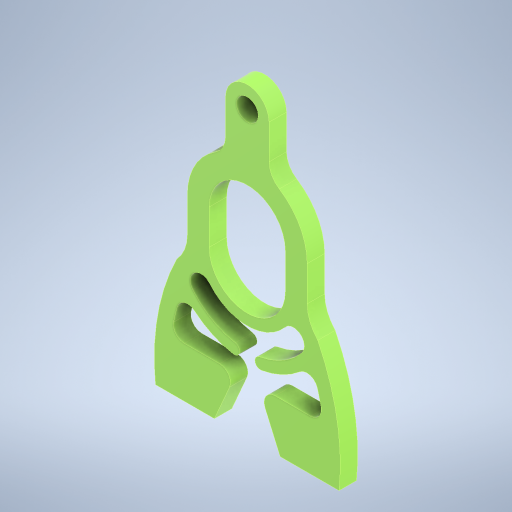
# Autodesk Inventor part: Back distributor
Saved by Autodesk Inventor 2023 (Build 270158000, 158)
## iProperties
Created: 2022-05-02
Part Number: Back distributor
Material: Phenolic Resin
Document SubType Name: Modeling
Designer: Devin
Density: 1.38 g/cm^3
Appearance: Light Green
Author: Devin
Autodesk Inventor part; units mm, degrees
ref_plane "YZ Plane" through (0, 0, 0) normal (1, 0, 0) x (0, 1, 0)
ref_plane "XZ Plane" through (0, 0, 0) normal (0, 1, 0) x (-1, 0, 0)
ref_plane "XY Plane" through (0, 0, 0) normal (0, 0, 1) x (1, 0, 0)
sketch "Sketch1" plane through (0, 0, 0) normal (0, 0, 1) x (1, 0, 0)
  circle A0 centre (0, 0) radius 1.27
  arc A1 (2.54, 0) -> (-2.54, 0) centre (0, 0) ccw
  line L0 (4.445, -12.065) -> (4.445, -16.129)
  line L1 (-4.445, -16.129) -> (-4.445, -12.065)
  arc A2 (-4.445, -16.129) -> (0, -20.574) centre (0, -16.129) ccw
  arc A3 (0, -20.574) -> (4.445, -16.129) centre (0, -16.129) ccw
  arc A4 (4.445, -12.065) -> (0, -7.62) centre (0, -12.065) ccw
  arc A5 (0, -7.62) -> (-4.445, -12.065) centre (0, -12.065) ccw
  arc A6 (-3.7253, -6.1564) -> (-6.985, -12.065) centre (0, -12.065) ccw
  line L2 (-6.985, -12.065) -> (-6.985, -16.129)
  line L3 (6.985, -16.129) -> (6.985, -12.065)
  arc A7 (6.985, -12.065) -> (3.7253, -6.1564) centre (0, -12.065) ccw
  line L4 (2.54, 0) -> (2.54, -4.0078)
  line L5 (-2.54, -4.0078) -> (-2.54, 0)
  arc A8 (-3.7253, -6.1564) -> (-2.54, -4.0078) centre (-5.08, -4.0078) ccw
  arc A9 (2.54, -4.0078) -> (3.7253, -6.1564) centre (5.08, -4.0078) ccw
  line L6 (0, 10.6389) -> (0, -34.9182) construction
  arc A10 (0, -21.844) -> (4.4127, -19.7607) centre (0, -16.129) ccw
  line L7 (5.715, -16.129) -> (5.715, -16.0811)
  arc A11 (-4.4127, -19.7607) -> (0, -21.844) centre (0, -16.129) ccw
  arc A12 (1.4151, -24.2618) -> (6.3739, -21.3748) centre (0, -16.129) ccw
  arc A13 (-6.3739, -21.3748) -> (-1.4151, -24.2618) centre (0, -16.129) ccw
  arc A14 (6.3739, -21.3748) -> (4.4127, -19.7607) centre (5.3933, -20.5678) ccw
  arc A15 (-4.4127, -19.7607) -> (-6.3739, -21.3748) centre (-5.3933, -20.5678) ccw
  arc A16 (-6.1402, -23.4108) -> (-1.6329, -25.513) centre (0, -16.129) ccw
  arc A17 (-1.6329, -25.513) -> (-1.4151, -24.2618) centre (-1.524, -24.8874) ccw
  arc A18 (1.4151, -24.2618) -> (1.6329, -25.513) centre (1.524, -24.8874) ccw
  arc A19 (-8.2215, -19.2053) -> (-6.985, -16.129) centre (-11.43, -16.129) ccw
  arc A20 (-8.2215, -19.2053) -> (-10.7047, -33.133) centre (14.5533, -30.451) ccw
  arc A21 (-8.1811, -24.0368) -> (-8.6001, -25.7693) centre (14.5533, -30.451) ccw
  arc A22 (6.985, -16.129) -> (8.2215, -19.2053) centre (11.43, -16.129) ccw
  arc A23 (10.7047, -33.133) -> (8.2215, -19.2053) centre (-14.5533, -30.451) ccw
  arc A24 (8.6001, -25.7693) -> (8.1811, -24.0368) centre (-14.5533, -30.451) ccw
  arc A25 (1.6329, -25.513) -> (6.1402, -23.4108) centre (0, -16.129) ccw
  line L8 (-3.8359, -33.133) -> (-2.0683, -29.0674)
  line L9 (3.8359, -33.133) -> (2.0683, -29.0674)
  line L10 (-7.3553, -27.291) -> (-3.2329, -27.291)
  line L11 (3.2329, -27.291) -> (7.3553, -27.291)
  line L12 (-10.7047, -33.133) -> (-3.8359, -33.133)
  line L13 (3.8359, -33.133) -> (10.7047, -33.133)
  arc A26 (-6.1402, -23.4108) -> (-8.1811, -24.0368) centre (-6.9589, -24.3817) ccw
  arc A27 (8.1811, -24.0368) -> (6.1402, -23.4108) centre (6.9589, -24.3817) ccw
  arc A28 (7.3553, -27.291) -> (8.6001, -25.7693) centre (7.3553, -26.021) ccw
  arc A29 (-8.6001, -25.7693) -> (-7.3553, -27.291) centre (-7.3553, -26.021) ccw
  arc A30 (-2.0683, -29.0674) -> (-3.2329, -27.291) centre (-3.2329, -28.561) ccw
  arc A31 (3.2329, -27.291) -> (2.0683, -29.0674) centre (3.2329, -28.561) ccw
  point P0 (4.445, -20.574)
  point P1 (4.445, -7.62)
  point P2 (-4.445, -20.574)
  point P3 (-2.54, -2.0039)
  point P4 (5.7149, -19.3392)
  point P5 (-5.7151, -19.3392)
  point P6 (-0.889, -24.8874)
  point P7 (0.889, -24.8874)
  point P8 (-10.7948, -28.8286)
  point P9 (10.7948, -28.8286)
  point P10 (-8.8563, -27.291)
  point P11 (8.8563, -27.291)
  point P12 (1.524, -25.5224)
  point P13 (-1.2959, -27.291)
  point P14 (1.2959, -27.291)
  point P15 (-4.4127, -19.7607)
  point P16 (0, -7.62)
  point P17 (0, -20.574)
  dimension "d0" = 2.54
  dimension "d1" = 1.27
  dimension "d2" = 8.89
  dimension "d3" = 12.954
  dimension "d4" = 4.445
  dimension "d5" = 2.54
  dimension "d8" = 2.54
  dimension "d10" = 4.0077
  dimension "d11" = 4.0077
  dimension "d13" = 1.27
  dimension "d14" = 2.54
  dimension "d15" = 11.43
  dimension "d18" = 1.27
  dimension "d19" = 1.778
  dimension "d27" = 1.778
  dimension "d33" = 2.54
  dimension "d34" = 5.842
  dimension "d37" = 1.27
  dimension "d38" = 1.27
  dimension "d39" = 1.27
  constraints: 72 point on circle, 32 centre point, 28 end point, 28 tangent, 9 point on line, 7 equal radius, 7 symmetric about line, 6 horizontal alignment, 4 horizontal, 3 parallel, 3 vertical, 2 coincident, 1 midpoint, 1 vertical alignment, 19 other
  measures "d0" diameter of A0
  measures "d1" radial gap between concentric circles of A0 A1
  measures "d2" distance of point (4.445, -20.574) point (-4.445, -20.574)
  measures "d3" distance of point (4.445, -7.62) point (4.445, -20.574)
  measures "d4" radius of A2
  measures "d5" radial gap between concentric circles of A4 A7
  measures "d8" radius of A8
  measures "d10" distance of L4.start L4.end
  measures "d11" distance of L5.start L5.end
  measures "d13" radial gap between concentric circles of A2 A11
  measures "d14" radial gap between concentric circles of A11 A13
  measures "d15" distance of point (5.715, -19.339) point (-5.715, -19.339)
  measures "d18" radial gap between concentric circles of A13 A16
  measures "d19" distance of point (0.889, -24.887) point (-0.889, -24.887)
  measures "d27" radial gap between concentric circles of A20 A21
  measures "d33" horizontal distance of L8.start point (-1.296, -27.291)
  measures "d34" distance between parallel lines of L12 L10
  measures "d37" radius of A26
  measures "d38" radius of A27
  measures "d39" radius of A30
extrude "Extrusion1" add sketch "Sketch1" along normal blind 2.032
body "Solid1"
